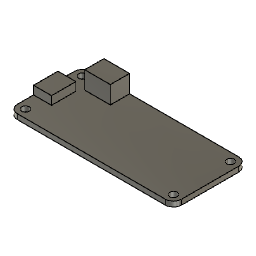
Wheel-Encoder-enclosure-short v4 (Autodesk Fusion 360 archive; units mm, degrees)
design "Feather BLE with Headers"
Autodesk Fusion 360 part; units mm, degrees
sketch "BLE" plane through (0, 0, 0) normal (0, 0, 1) x (1, 0, 0) in component "Part 1 v1"
  line L0 (51.2, 0) -> (51.2, 22.86)
  line L1 (51.2, 22.86) -> (0, 22.86)
  line L2 (0, 22.86) -> (0, 0)
  line L3 (0, 0) -> (51.2, 0)
  circle A0 centre (48.66, 20.32) radius 1.2
  circle A1 centre (48.66, 2.54) radius 1.2
  circle A2 centre (2.54, 20.32) radius 1.2
  circle A3 centre (2.54, 2.54) radius 1.2
  line L4 (5.6, 7.6) -> (5.6, 15.2)
  line L5 (5.6, 15.2) -> (0, 15.2)
  line L6 (0, 15.2) -> (0, 7.6)
  line L7 (0, 7.6) -> (5.6, 7.6)
  line L8 (5.6, 7.6) -> (0, 15.2) construction
  line L9 (5.6, 15.2) -> (0, 7.6) construction
  line L10 (6.668, 22.86) -> (6.668, 16.86)
  line L11 (6.668, 16.86) -> (14.668, 16.86)
  line L12 (14.668, 16.86) -> (14.668, 22.86)
  line L13 (14.668, 22.86) -> (6.668, 22.86)
  line L14 (6.668, 22.86) -> (14.668, 16.86) construction
  line L15 (6.668, 16.86) -> (14.668, 22.86) construction
  point P0 (25.6, 11.4)
  point P1 (2.8, 11.4)
  point P2 (10.668, 19.86)
  dimension "d11" = 22.86
  dimension "d12" = 51.2
  dimension "d13" = 2.4
  dimension "d14" = 2.54
  dimension "d15" = 2.54
  dimension "d16" = 7.6
  dimension "d17" = 5.6
  dimension "d18" = 6
  dimension "d19" = 8
  dimension "d20" = 10.668
  dimension "d30" = 2.54
  dimension "d31" = 2.54
  dimension "d32" = 2.54
  dimension "d33" = 2.54
  dimension "d34" = 2.54
  dimension "d35" = 2.54
  constraint perpendicular L0 L1
  constraint parallel L0 L2
  constraint parallel L1 L3
  constraint perpendicular L4 L5
  constraint parallel L4 L6
  constraint parallel L5 L7
  constraint coincident L8 P1
  constraint coincident L9 P1
  constraint collinear L2 L6
  constraint perpendicular L10 L11
  constraint parallel L10 L12
  constraint parallel L11 L13
  constraint coincident L14 P2
  constraint coincident L15 P2
  constraint collinear L1 L13
  constraint coincident L2.end L3.start
  measures "d11" distance of L1.end L2.end
  measures "d12" distance of L0.end L1.end
  measures "d13" diameter of A0
  measures "d14" distance of L0 A0.centre
  measures "d15" distance of L1 A0.centre
  measures "d16" distance of L5.end L6.end
  measures "d17" distance of L4.end L5.end
  measures "d18" distance of L11.end L12.end
  measures "d19" distance of L10.end L11.end
  measures "d20" distance of L2 P2
  measures "d30" distance of L2 A3.centre
  measures "d31" distance of L3 A3.centre
  measures "d32" distance of L2 A2.centre
  measures "d33" distance of L1 A2.centre
  measures "d34" distance of L3 A1.centre
  measures "d35" distance of L0 A1.centre
extrude "Extrude3" add sketch "BLE" along normal blind 1.6 makes body 1 in component "Part 1 v1"
extrude "Extrude4" add sketch "BLE" along normal blind 7.1 and the other way blind -1.6 separate body contours L1 L10 L11 L12 L13 makes body 2 in component "Part 1 v1"
extrude "Extrude5" add sketch "BLE" along normal blind 4.2 and the other way blind -1.6 separate body contours L2 L4 L5 L6 L7 makes body 3 in component "Part 1 v1"
fillet "Fillet1" radius 2.54 4 edges at (0, 22.86, 0.8) (0, 0, 0.8) (51.2, 0, 0.8) (51.2, 22.86, 0.8) on bodies 1 in component "Part 1 v1"
sketch "headers" plane through (0, 0, 0) normal (0, 0, -1) x (1, 0, 0)
  circle A0 centre (48.66, -2.54) radius 1.2
  circle A1 centre (2.54, -20.32) radius 1.2
  circle A2 centre (2.54, -2.54) radius 1.2
  circle A3 centre (48.66, -20.32) radius 1.2
  arc A4 (48.66, -22.86) -> (51.2, -20.32) centre (48.66, -20.32) ccw
  line L0 (51.2, -20.32) -> (51.2, -2.54)
  arc A5 (51.2, -2.54) -> (48.66, 0) centre (48.66, -2.54) ccw
  line L1 (48.66, 0) -> (2.54, 0)
  arc A6 (2.54, 0) -> (0, -2.54) centre (2.54, -2.54) ccw
  line L2 (0, -2.54) -> (0, -20.32)
  arc A7 (0, -20.32) -> (2.54, -22.86) centre (2.54, -20.32) ccw
  line L3 (2.54, -22.86) -> (48.66, -22.86)
  line L4 (6.2, 0) -> (46.2, 0)
  line L5 (46.2, 0) -> (46.2, -2.5)
  line L6 (46.2, -2.5) -> (6.2, -2.5)
  line L7 (6.2, -2.5) -> (6.2, 0)
  line L8 (46.2, -22.86) -> (15.2, -22.86)
  line L9 (15.2, -22.86) -> (15.2, -20.36)
  line L10 (15.2, -20.36) -> (46.2, -20.36)
  line L11 (46.2, -20.36) -> (46.2, -22.86)
  dimension "d5" = 40
  dimension "d6" = 2.5
  dimension "d8" = 31
  dimension "d9" = 2.5
  dimension "d10" = 5
  dimension "d36" = 5
  constraint horizontal L4
  constraint vertical L5
  constraint horizontal L6
  constraint vertical L7
  constraint collinear L1 L4
  constraint horizontal L8
  constraint vertical L9
  constraint horizontal L10
  constraint vertical L11
  constraint collinear L3 L8
  measures "d5" distance of L4.start L4.end
  measures "d6" distance of L4.start L6.end
  measures "d8" distance of L8.start L8.end
  measures "d9" distance of L8.start L10.end
  measures "d10" distance of L0 L11
  measures "d36" distance of L0 L5
extrude "Extrude1" [rolled back] along distance 7.6 taper angle 0
move_body "Move1" [rolled back]
component "Part 1 v1" placed x (1, 0, 0) y (0, 1, 0) z (0, 0, 1) at (0, 0, 0)
equation "d23 = 5.5 mm + 1.6 mm"
named bodies: "feather BLE pcb", "jst", "microUSB", "header 12x", "header 16x"
